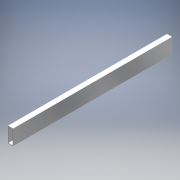
# Autodesk Inventor part: Back Extrusion
Saved by Autodesk Inventor 2019.4 (Build 234330000, 330)
## iProperties
Created: 2020-01-05
Part Number: Back Extrusion
Material: Aluminum 6061
Document SubType Name: Modeling
Designer: Mark
Mass: 517.104 g
Surface Area: 1921.28 cm^2
Volume: 191.52 cm^3
Density: 2.7 g/cm^3
Appearance: Aluminum - Flat
Author: Mark
Autodesk Inventor part; units mm, degrees
ref_plane "YZ Plane" through (0, 0, 0) normal (1, 0, 0) x (0, 1, 0)
ref_plane "XZ Plane" through (0, 0, 0) normal (0, 1, 0) x (-1, 0, 0)
ref_plane "XY Plane" through (0, 0, 0) normal (0, 0, 1) x (1, 0, 0)
sketch "Sketch1" plane through (0, 0, 0) normal (0, 0, 1) x (1, 0, 0)
  line L0 (-10, -30) -> (10, -30)
  line L1 (10, -30) -> (10, 30)
  line L2 (10, 30) -> (-10, 30)
  line L3 (-10, 30) -> (-10, -30)
  line L4 (-10, -30) -> (10, 30) construction
  line L5 (10, -30) -> (-10, 30) construction
  line L6 (8, -28) -> (-8, -28)
  line L7 (-8, -28) -> (-8, 28)
  line L8 (-8, 28) -> (8, 28)
  line L9 (8, 28) -> (8, -28)
  line L10 (8, -28) -> (-8, 28) construction
  line L11 (-8, -28) -> (8, 28) construction
  point P0 (0, 0)
  dimension "d0" = 20
  dimension "d1" = 60
  dimension "d2" = 16
  dimension "d3" = 56
  constraints: 24 end point, 4 midpoint, 4 parallel, 2 horizontal, 2 perpendicular
  measures "d0" distance of L2.end L1.end
  measures "d1" distance of L1.end L0.end
  measures "d2" distance of L7.end L8.end
  measures "d3" distance of L6.end L7.end
extrude "Extrusion1" add sketch "Sketch1" along normal blind 570
body "Solid1"
